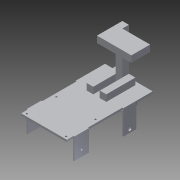
# Autodesk Inventor part: robot chasis
Saved by Autodesk Inventor 2014 (Build 180170000, 170)
## iProperties
Created: 2014-11-30
Part Number: robot chasis
Material: Generic
Document SubType Name: Modeling
Designer: ph1140784
Density: 1 g/cm^3
Appearance: Aluminum - Flat
Author: ph1140784
Autodesk Inventor part; units mm, degrees
ref_plane "YZ Plane" through (0, 0, 0) normal (1, 0, 0) x (0, 1, 0)
ref_plane "XZ Plane" through (0, 0, 0) normal (0, 1, 0) x (-1, 0, 0)
ref_plane "XY Plane" through (0, 0, 0) normal (0, 0, 1) x (1, 0, 0)
sketch "Sketch2" plane through (0, 0, 0) normal (0, 1, 0) x (-1, 0, 0)
  line L0 (-25.5, 14.5) -> (-5.5, 14.5)
  line L1 (-5.5, 14.5) -> (-5.5, -5.5)
  line L2 (-5.5, -5.5) -> (-25.5, -5.5)
  line L3 (-25.5, -5.5) -> (-25.5, 14.5)
  line L4 (-25.5, 14.5) -> (-5.5, -5.5) construction
  line L5 (-5.5, 14.5) -> (-25.5, -5.5) construction
  point P0 (0, 0)
  point P1 (-15.5, 4.5)
  dimension "d0" = 20
  dimension "d1" = 20
  constraints: 12 end point, 2 midpoint, 2 parallel, 1 horizontal, 1 perpendicular
  measures "d0" distance of L1.end L2.end
  measures "d1" distance of L0.end L1.end
extrude "Extrusion1" add sketch "Sketch2" along normal blind 210
sketch "Sketch3" plane through (25.5, 0, 14.5) normal (1, 0, 0) x (0, 0, -1)
  line L0 (20, 0) -> (20, 210) projected
  line L1 (0, 137.5) -> (20, 137.5)
  line L2 (20, 137.5) -> (20, 117.5)
  line L3 (20, 117.5) -> (0, 117.5)
  line L4 (0, 117.5) -> (0, 137.5)
  line L5 (0, 137.5) -> (20, 117.5) construction
  line L6 (20, 137.5) -> (0, 117.5) construction
  point P0 (14.5, 0)
  point P1 (10, 127.5)
  dimension "d4" = 20
  constraints: 12 end point, 2 midpoint, 2 parallel, 1 horizontal, 1 perpendicular, 1 point on line
  measures "d4" distance of L1.end L2.end
extrude "Extrusion2" add sketch "Sketch3" along normal blind 100
ref_plane "Work Plane1" through (75.5, 0, 14.5) normal (1, 0, 0) x (0, 0, -1)
mirror "Mirror1" about plane through (75.5, 0, 14.5) normal (1, 0, 0) of "Extrusion1"
sketch "Sketch4" plane through (5.5, 0, 14.5) normal (0, 0, 1) x (1, 0, 0)
  line L0 (60, 250) -> (80, 250)
  line L1 (80, 250) -> (80, 230)
  line L2 (80, 230) -> (60, 230)
  line L3 (60, 230) -> (60, 250)
  line L4 (60, 250) -> (80, 230) construction
  line L5 (80, 250) -> (60, 230) construction
  point P0 (-5.5, 0)
  point P1 (20, 112.5)
  point P2 (70, 240)
  constraints: 12 end point, 2 parallel, 1 horizontal, 1 perpendicular
extrude "Extrusion3" add sketch "Sketch4" along normal blind 150
sketch "Sketch11" plane through (5.5, 0, 14.5) normal (0, 0, 1) x (1, 0, 0)
  circle A0 centre (10, 8) radius 2.5
  circle A1 centre (10, 98) radius 2.5
  circle A2 centre (130, 8) radius 2.5
  circle A3 centre (130, 98) radius 2.5
  point P0 (-5.5, 0)
  dimension "d25" = 5
  dimension "d28" = 90
  dimension "d31" = 120
  dimension "d39" = 120
  constraints: 4 centre point
  measures "d25" diameter of A0
  measures "d28" distance of A0.centre A1.centre
  measures "d31" distance of A0.centre A2.centre
  measures "d39" distance of A3.centre A1.centre
extrude "Extrusion10" cut sketch "Sketch11" against normal blind 36
sketch "Sketch13" plane through (5.5, 0, 14.5) normal (0, 0, 1) x (1, 0, 0)
  circle A0 centre (130, 8) radius 2.5 projected
  circle A1 centre (10, 8) radius 2.5 projected
  circle A2 centre (10, 98) radius 2.5 projected
  circle A3 centre (130, 98) radius 2.5 projected
  line L0 (0, 110) -> (150, 110)
  line L1 (0, 110) -> (0, 0)
  line L2 (0, 0) -> (150, 0)
  line L3 (150, 0) -> (150, 110)
  line L4 (0, 110) -> (0, 55)
  line L5 (0, 55) -> (150, 55)
  point P0 (-5.5, 0)
  dimension "d36" = 55
  constraints: 12 end point, 2 midpoint, 2 perpendicular, 1 parallel
  measures "d36" distance of L0.start L4.end
sketch "Sketch14" plane through (145.5, 0, 14.5) normal (1, 0, 0) x (0, 0, -1)
  line L0 (0, 20) -> (65, 20)
  line L1 (65, 20) -> (65, 65)
  line L2 (65, 65) -> (0, 65)
  line L3 (0, 65) -> (0, 20)
  circle A0 centre (45, 42.5) radius 3.5
  dimension "d44" = 7
  dimension "d45" = 20
  constraints: 8 end point, 2 parallel, 1 centre point, 1 horizontal, 1 perpendicular
  measures "d44" diameter of A0
  measures "d45" horizontal distance of L0.end A0.centre
ref_plane "Work Plane2" through (75.5, 250, 14.5) normal (1, 0, 0) x (0, 0, -1)
extrude "Extrusion12" add sketch "Sketch14" along normal blind 3
mirror "Mirror3" about plane through (75.5, 250, 14.5) normal (1, 0, 0) of "Extrusion12"
sketch "Sketch15" plane through (5.5, 0, 14.5) normal (0, 0, 1) x (1, 0, 0)
  line L0 (0, 0) -> (0, 20) projected
  line L1 (20, 0) -> (0, 0) projected
  line L2 (0, 0) -> (140, 0)
  line L3 (140, 0) -> (140, 110)
  line L4 (0, 110) -> (0, 0)
  line L5 (0, 110) -> (140, 110)
  circle A0 centre (10, 98) radius 2.5 projected
  circle A1 centre (10, 8) radius 2.5 projected
  circle A2 centre (130, 98) radius 2.5 projected
  circle A3 centre (130, 8) radius 2.5 projected
  point P0 (-5.5, 0)
  constraints: 8 end point, 2 perpendicular, 1 horizontal, 1 parallel
sketch "Sketch18" plane through (5.5, 210, -5.5) normal (-1, 0, 0) x (0, 0, 1)
  line L0 (20, 0) -> (-55, 0)
  line L1 (-55, 0) -> (-55, -40)
  line L2 (-55, -40) -> (20, -40)
  line L3 (20, -40) -> (20, 0)
  point P0 (5.5, -210)
  point P1 (-45, -20)
  dimension "d51" = 75
  constraints: 8 end point, 2 parallel, 1 horizontal, 1 perpendicular
  measures "d51" distance of L2.end L1.end
extrude "Extrusion13" add sketch "Sketch18" along normal blind 3
mirror "Mirror4" about plane through (75.5, 250, 14.5) normal (1, 0, 0) of "Extrusion13"
sketch "Sketch19" plane through (2.5, 210, -5.5) normal (-1, 0, 0) x (0, 0, 1)
  line L0 (-55, 0) -> (-55, -40) projected
  circle A0 centre (-45, -20) radius 5
  point P0 (5.5, -210)
  dimension "d54" = 10
  dimension "d55" = 10
  constraints: 1 centre point
  measures "d54" diameter of A0
  measures "d55" distance from line of L0 A0.centre
extrude "Extrusion14" cut sketch "Sketch19" against normal through all
sketch "Sketch20" plane through (25.5, 0, 14.5) normal (1, 0, 0) x (0, 0, -1)
  line L0 (20, 117.5) -> (0, 117.5) projected
  line L1 (0, 0) -> (0, 117.5) projected
  line L2 (20, 0) -> (0, 0) projected
  line L3 (0, 0) -> (0, 117.5)
  line L4 (6, 117.5) -> (6, 0)
  line L5 (0, 137.5) -> (0, 210) projected
  line L6 (0, 210) -> (20, 210) projected
  line L7 (6, 210) -> (6, 137.5)
  line L8 (6, 137.5) -> (0, 137.5)
  point P0 (14.5, 0)
  constraints: 8 end point, 3 point on line, 2 perpendicular, 1 collinear, 1 parallel
extrude "Extrusion15" add sketch "Sketch20" along normal up to next
sketch "Sketch21" plane through (0, 0, 0) normal (0, -1, 0) x (1, 0, 0)
  line L0 (145.5, 14.5) -> (145.5, -5.5) projected
  line L1 (5.5, -5.5) -> (145.5, -5.5)
  line L2 (145.5, -5.5) -> (145.5, 8.5)
  line L3 (145.5, 8.5) -> (5.5, 8.5)
  line L4 (5.5, 8.5) -> (5.5, -5.5)
  point P0 (0, 0)
  constraints: 8 end point, 2 parallel, 1 horizontal, 1 perpendicular, 1 point on line
extrude "Extrusion16" cut sketch "Sketch21" against normal through all
sketch "Sketch22" plane through (145.5, 210, 8.5) normal (0, 0, -1) x (-1, 0, 0)
  line L0 (0, 0) -> (140, 0) projected
  line L1 (70, 50) -> (45, 50)
  line L2 (70, 50) -> (95, 50)
  line L3 (70, 30) -> (82.5, 30)
  line L4 (82.5, 30) -> (70, 30)
  line L5 (82.5, 30) -> (95, 50)
  line L6 (57.5, 30) -> (70, 30)
  line L7 (57.5, 30) -> (45, 50)
  point P0 (145.5, -210)
  point P1 (70, 50)
  constraints: 14 end point, 1 collinear
extrude "Extrusion17" add sketch "Sketch22" along normal blind 3
sketch "Sketch25" plane through (0, 210, 0) normal (0, 1, 0) x (1, 0, 0)
  line L0 (145.5, -8.5) -> (5.5, -8.5) projected
  line L1 (148.5, -14.5) -> (148.5, 60.5) projected
  line L2 (2.5, -14.5) -> (148.5, -14.5)
  line L3 (148.5, -14.5) -> (148.5, -8.5)
  line L4 (148.5, -8.5) -> (2.5, -8.5)
  line L5 (2.5, -8.5) -> (2.5, -14.5)
  point P0 (100.5, -8.5)
  point P1 (0, 0)
  constraints: 8 end point, 2 parallel, 2 point on line, 1 horizontal, 1 perpendicular
extrude "Extrusion20" add sketch "Sketch25" along normal blind 50
sketch "Sketch26" plane through (145.5, 210, 5.5) normal (0, 0, -1) x (-1, 0, 0)
  line L0 (95, 50) -> (45, 50) projected
  line L1 (45, 50) -> (57.5, 30) projected
  line L2 (57.5, 30) -> (82.5, 30) projected
  line L3 (82.5, 30) -> (95, 50) projected
  line L4 (46.875, 47) -> (93.125, 47)
  point P0 (145.5, -210)
  dimension "d73" = 3
  constraints: 2 end point, 2 point on line, 1 parallel
  measures "d73" vertical distance of L4.end L0.start
extrude "Extrusion21" add sketch "Sketch26" along normal blind 50 contours L3 L4 L1 L0
sketch "Sketch27" plane through (52.375, 257, 5.5) normal (0, -1, 0) x (1, 0, 0)
  line L0 (46.25, 0) -> (46.25, -50) projected
  line L1 (0, -50) -> (46.25, -50)
  line L2 (46.25, -50) -> (46.25, -47)
  line L3 (46.25, -47) -> (0, -47)
  line L4 (0, -47) -> (0, -50)
  point P0 (-52.375, -5.5)
  constraints: 8 end point, 2 parallel, 1 horizontal, 1 perpendicular, 1 point on line
extrude "Extrusion22" add sketch "Sketch27" along normal blind 40
sketch "Sketch28" plane through (5.5, 0, 14.5) normal (0, 0, 1) x (1, 0, 0)
  line L0 (60, 250) -> (40, 250)
  line L1 (40, 250) -> (40, 161)
  line L2 (40, 161) -> (60, 161)
  line L3 (60, 161) -> (60, 250)
  line L4 (80, 250) -> (100, 250)
  line L5 (100, 250) -> (100, 161)
  line L6 (100, 161) -> (80, 161)
  line L7 (80, 161) -> (80, 250)
  point P0 (-5.5, 0)
  constraints: 16 end point, 4 parallel, 2 horizontal, 2 perpendicular
extrude "Extrusion23" add sketch "Sketch28" along normal blind 20
ref_plane "Work Plane3" through (85.5, 117.5, 14.5) normal (-1, 0, 0) x (0, 0, 1)
sketch "Sketch29" plane through (85.5, 117.5, 14.5) normal (-1, 0, 0) x (0, 0, 1)
  line L0 (130, 112.5) -> (150, 112.5) projected
  line L1 (130, 112.5) -> (130, 55) projected
  line L2 (130, 55) -> (150, 55) projected
  line L3 (150, 55) -> (150, 112.5) projected
  point P0 (-14.5, -117.5)
extrude "Extrusion24" add sketch "Sketch29" along normal blind 20
ref_plane "Work Plane4" through (170.5, 117.5, 14.5) normal (1, 0, 0) x (0, 0, -1)
sketch "Sketch32" plane through (85.5, 230, 34.5) normal (1, 0, 0) x (0, 0, -1)
  line L0 (-130, -57.5) -> (-130, 20) projected
  line L1 (-110, -57.5) -> (-130, -57.5) projected
  line L2 (-110, 0) -> (-110, -57.5) projected
  line L3 (0, 0) -> (-110, 0) projected
  line L4 (-130, 0) -> (-110, 0)
  point P0 (34.5, -230)
  constraints: 3 end point, 1 point on line
extrude "Extrusion26" add sketch "Sketch32" along normal blind 85
body "Solid1"
